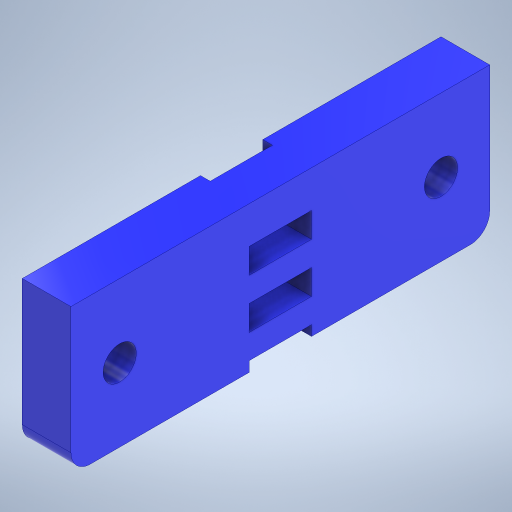
# Autodesk Inventor part: RZvector-v1-Plate-B-F
Saved by Autodesk Inventor 2024.1 (Build 281209000, 209)
## iProperties
Created: 2024-03-12
Part Number: RZvector-v1-Plate-B-F
Material: ABS プラスチック
Document SubType Name: Modeling
Designer: haruy
Density: 1.06 g/cm^3
Appearance: 青 - 壁塗料 - 光沢
Author: haruy
Autodesk Inventor part; units mm, degrees
ref_plane "YZ Plane" through (0, 0, 0) normal (1, 0, 0) x (0, 1, 0)
ref_plane "XZ Plane" through (0, 0, 0) normal (0, 1, 0) x (-1, 0, 0)
ref_plane "XY Plane" through (0, 0, 0) normal (0, 0, 1) x (1, 0, 0)
sketch "スケッチ1" plane through (0, 0, 0) normal (1, 0, 0) x (0, 1, 0)
  line L0 (0, 0) -> (30, 0)
  line L1 (30, 0) -> (30, -43)
  line L2 (30, -43) -> (0, -43)
  line L3 (0, -43) -> (0, 0)
  circle A0 centre (15, -5) radius 1.5
  circle A1 centre (15, -38) radius 1.5
  line L4 (30, -21.5) -> (0, -21.5)
  line L5 (30, -18.3) -> (0, -18.3)
  line L6 (30, -24.7) -> (0, -24.7)
  line L7 (15, 0) -> (15, -43)
  line L8 (16.285, -18.3) -> (16.285, -24.7)
  line L9 (13.715, -18.3) -> (13.715, -24.7)
  line L10 (20.08, -18.3) -> (20.08, -24.7)
  line L11 (25.16, -18.3) -> (25.16, -24.7)
  line L12 (30.24, -18.3) -> (30.24, -24.7)
  line L13 (21.365, -18.3) -> (21.365, -24.7)
  line L14 (26.445, -18.3) -> (26.445, -24.7)
  line L15 (28.955, -18.3) -> (28.955, -24.7)
  line L16 (23.875, -18.3) -> (23.875, -24.7)
  line L17 (18.795, -18.3) -> (18.795, -24.7)
  line L18 (8.635, -18.3) -> (8.635, -24.7)
  line L19 (3.555, -18.3) -> (3.555, -24.7)
  line L20 (1.045, -18.3) -> (1.045, -24.7)
  line L21 (6.125, -18.3) -> (6.125, -24.7)
  line L22 (11.205, -18.3) -> (11.205, -24.7)
  circle A2 centre (7.5, -5) radius 1.7
  circle A3 centre (22.5, -5) radius 1.7
  circle A4 centre (22.5, -38) radius 1.7
  circle A5 centre (7.5, -38) radius 1.7
  point P0 (15, -24.7)
  point P1 (15, -18.3)
  dimension "d0" = 30
  dimension "d1" = 43
  dimension "d2" = 3
  dimension "d3" = 3
  dimension "d4" = 5
  dimension "d5" = 5
  dimension "d6" = 15
  dimension "d7" = 15
  dimension "d8" = 3.2
  dimension "d9" = 3.2
  dimension "d10" = 1.285
  dimension "d11" = 1.285
  dimension "d12" = 5.08
  dimension "d13" = 5.08
  dimension "d14" = 5.08
  dimension "d15" = 1.285
  dimension "d16" = 1.285
  dimension "d17" = 1.285
  dimension "d21" = 3.4
  dimension "d22" = 3.4
  dimension "d23" = 3.4
  dimension "d24" = 3.4
  dimension "d25" = 5
  dimension "d26" = 5
  dimension "d27" = 7.5
  dimension "d28" = 7.5
  dimension "d29" = 7.5
  dimension "d30" = 5
  dimension "d31" = 7.5
  dimension "d32" = 5
  constraints: 42 end point, 14 symmetric about line, 9 vertical, 6 centre point, 4 midpoint, 4 point on line, 3 parallel, 1 horizontal, 1 perpendicular, 20 other
  measures "d0" distance of L1.end L2.end
  measures "d1" distance of L0.end L1.end
  measures "d2" diameter of A0
  measures "d3" diameter of A1
  measures "d4" distance from line of L0 A0.centre
  measures "d5" distance from line of A1.centre L2
  measures "d6" distance from line of A0.centre L3
  measures "d7" distance from line of A1.centre L3
  measures "d10" distance between parallel lines of L7 L8
  measures "d11" distance between parallel lines of L9 L7
  measures "d12" distance between parallel lines of L7 L10
  measures "d13" distance between parallel lines of L10 L11
  measures "d14" distance between parallel lines of L11 L12
  measures "d15" distance between parallel lines of L10 L13
  measures "d16" distance between parallel lines of L11 L14
  measures "d17" distance between parallel lines of L15 L12
  measures "d21" diameter of A2
  measures "d22" diameter of A3
  measures "d23" diameter of A4
  measures "d24" diameter of A5
  measures "d25" distance from line of A2.centre L0
  measures "d26" distance from line of A3.centre L0
  measures "d27" distance from line of A2.centre L3
  measures "d28" distance from line of A3.centre L1
  measures "d29" distance from line of A5.centre L3
  measures "d30" distance from line of L2 A5.centre
  measures "d31" distance from line of A4.centre L1
  measures "d32" distance from line of L2 A4.centre
extrude "押し出し1" add sketch "スケッチ1" along normal blind 4 contours L0 L7 A0 L5 L3 | L7 A0 | L5 L19 L4 L20 | L6 L7 A1 L2 L3 | L4 L19 L6 L20 | L7 L4 L9 L5 | L5 L18 L4 L21 | L9 L4 L22 L5 | L7 L6 L9 L4 | L4 L18 L6 L21 | L9 L6 L22 L4 | A1 L7 picked at (14.3164, -4.583) picked at (14.3492, -38.284)
sketch "スケッチ2" plane through (4, 0, 0) normal (1, 0, 0) x (0, 0, -1)
  line L0 (24.7, 1.045) -> (24.7, 0) projected
  line L1 (18.3, 0) -> (18.3, 1.045) projected
  line L2 (0, 15) -> (0, 0) projected
  line L3 (0, 0) -> (18.3, 0) projected
  line L4 (18.3, 1.045) -> (24.7, 1.045) projected
  line L5 (24.7, 0) -> (43, 0) projected
  line L6 (43, 0) -> (43, 15) projected
  line L7 (18.3, 3.555) -> (18.3, 6.125) projected
  line L8 (18.3, 6.125) -> (24.7, 6.125) projected
  line L9 (24.7, 6.125) -> (24.7, 3.555) projected
  line L10 (24.7, 3.555) -> (18.3, 3.555) projected
  line L11 (18.3, 11.205) -> (24.7, 11.205) projected
  line L12 (24.7, 11.205) -> (24.7, 8.635) projected
  line L13 (24.7, 8.635) -> (18.3, 8.635) projected
  line L14 (18.3, 8.635) -> (18.3, 11.205) projected
  line L15 (43, 15) -> (0, 15) projected
extrude "押し出し2" add sketch "スケッチ1" against normal blind 1 contours L0 L7 A0 L5 L3 | L7 A0 | L6 L7 A1 L2 L3 | A1 L7 picked at (14.3164, -4.583) picked at (14.3492, -38.284)
fillet "フィレット2" radius 2 2 edges at (1.5, 0, 0) (1.5, 0, -43)
